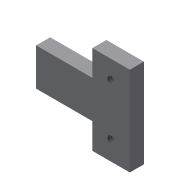
# Autodesk Inventor part: Tbracket
Saved by Autodesk Inventor 2022 (Build 260148000, 148)
## iProperties
Created: 2006-01-12
Part Number: Tbracket
Document SubType Name: Modeling
Designer: Administrator
Density: 1 g/cm^3
Material: Generic
Appearance: Default
Author: Administrator
Autodesk Inventor part; units mm, degrees
ref_plane "YZ Plane" through (0, 0, 0) normal (1, 0, 0) x (0, 1, 0)
ref_plane "XZ Plane" through (0, 0, 0) normal (0, 1, 0) x (-1, 0, 0)
ref_plane "XY Plane" through (0, 0, 0) normal (0, 0, 1) x (1, 0, 0)
sketch "Sketch1" plane through (0, 0, 0) normal (0, 0, 1) x (1, 0, 0)
  line L0 (0, 0) -> (-127, 0) projected
  line L1 (0, 0) -> (0, 25.4) projected
  line L2 (0, 25.4) -> (-127, 25.4) projected
  line L3 (-127, 0) -> (-127, 25.4) projected
  line L4 (0, 73.025) -> (-50.8, 73.025)
  line L5 (-50.8, 73.025) -> (-50.8, -47.625)
  line L6 (-50.8, -47.625) -> (0, -47.625)
  line L7 (0, -47.625) -> (0, 73.025)
  line L8 (-50.8, 38.1) -> (-127, 38.1)
  line L9 (-127, 38.1) -> (-127, -12.7)
  line L10 (-127, -12.7) -> (-50.8, -12.7)
  line L11 (-50.8, -12.7) -> (-50.8, 38.1)
  line L12 (-150.4488, 12.7) -> (41.0315, 12.7)
  dimension "d0" = 50.8
  dimension "d1" = 0
  dimension "d2" = 50.8
  dimension "d4" = 120.65
  dimension "d5" = 60.325
  dimension "d6" = 25.4
  constraints: 18 end point, 4 parallel, 3 horizontal, 2 perpendicular, 1 collinear, 1 point on line, 2 other
  measures "d0" distance of L5.end L6.end
  measures "d1" distance between parallel lines of L7 L1
  measures "d2" distance of L8.end L9.end
  measures "d4" distance of L6.end L4.start
  measures "d5" distance between parallel lines of L4 L12
  measures "d6" distance between parallel lines of L12 L10
extrude "Extrusion1" add sketch "Sketch1" along normal blind 19.05
hole "Hole1" at (-25.4, 47.625, 19.05) direction (0, 0, -1) diameter 10.5918 end through all thread size "1/2-13 UNC" class "1B" standard "ANSI Unified Screw Threads"
hole "Hole2" at (-25.4, -22.225, 19.05) direction (0, 0, -1) diameter 10.5918 end through all thread size "1/2-13 UNC" class "1B" standard "ANSI Unified Screw Threads"
equation "\"d2\" = d0"
equation "\"d5\" = 0.5 * d4"
equation "\"d6\" = 0.5 * d2"
body "Solid1"
